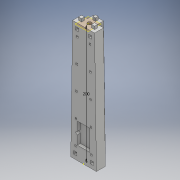
# Autodesk Inventor part: tb3_pt3
Saved by Autodesk Inventor 2017 (Build 210142000, 142)
## iProperties
Created: 2017-04-07
Part Number: tb3_pt3
Material: Generic
Document SubType Name: Modeling
Designer: PC
Density: 1 g/cm^3
Appearance: Default
Author: PC
Autodesk Inventor part; units mm, degrees
ref_plane "YZ Plane" through (0, 0, 0) normal (1, 0, 0) x (0, 1, 0)
ref_plane "XZ Plane" through (0, 0, 0) normal (0, 1, 0) x (-1, 0, 0)
ref_plane "XY Plane" through (0, 0, 0) normal (0, 0, 1) x (1, 0, 0)
sketch "Sketch1" plane through (0, 0, 0) normal (0, 0, 1) x (1, 0, 0)
  line L0 (21.5, -7.5) -> (-21.5, -7.5)
  line L1 (-21.5, -7.5) -> (-21.5, 7.5)
  line L2 (-21.5, 7.5) -> (21.5, 7.5)
  line L3 (21.5, 7.5) -> (21.5, -7.5)
  line L4 (21.5, -7.5) -> (-21.5, 7.5) construction
  line L5 (-21.5, -7.5) -> (21.5, 7.5) construction
  point P0 (0, 0)
  dimension "d0" = 43
  dimension "d1" = 15
  constraints: 12 end point, 2 midpoint, 2 parallel, 1 horizontal, 1 perpendicular
  measures "d0" distance of L1.end L2.end
  measures "d1" distance of L0.end L1.end
sketch "Sketch2" plane through (0, 0, 0) normal (0, 0, 1) x (1, 0, 0)
  line L0 (0, 0) -> (0, 12.5)
  line L1 (11.5, 17.5) -> (-11.5, 17.5)
  line L2 (-11.5, 17.5) -> (-11.5, 7.5)
  line L3 (-11.5, 7.5) -> (11.5, 7.5)
  line L4 (11.5, 7.5) -> (11.5, 17.5)
  line L5 (11.5, 17.5) -> (-11.5, 7.5) construction
  line L6 (-11.5, 17.5) -> (11.5, 7.5) construction
  dimension "d2" = 12.5
  dimension "d3" = 23
  dimension "d4" = 10
  constraints: 14 end point, 2 midpoint, 2 parallel, 1 horizontal, 1 perpendicular, 1 vertical
  measures "d2" distance of L0.start L0.end
  measures "d3" distance of L3.end L2.end
  measures "d4" distance of L2.end L1.end
sketch "Sketch3" plane through (0, 0, 0) normal (1, 0, 0) x (0, 1, 0)
  line L0 (0, 0) -> (0, 200)
  dimension "d5" = 200
  constraints: 2 end point, 1 vertical
  measures "d5" distance of L0.start L0.end
ref_plane "Work Plane1" through (0, 0, 200) normal (0, 0, 1) x (1, 0, 0)
sketch "Sketch4" plane through (0, 0, 200) normal (0, 0, 1) x (1, 0, 0)
  line L0 (18.5, -7.5) -> (-18.5, -7.5)
  line L1 (-18.5, -7.5) -> (-18.5, 7.5)
  line L2 (-18.5, 7.5) -> (18.5, 7.5)
  line L3 (18.5, 7.5) -> (18.5, -7.5)
  line L4 (18.5, -7.5) -> (-18.5, 7.5) construction
  line L5 (-18.5, -7.5) -> (18.5, 7.5) construction
  point P0 (0, 0)
  dimension "d6" = 37
  dimension "d7" = 15
  constraints: 12 end point, 2 midpoint, 2 parallel, 1 horizontal, 1 perpendicular
  measures "d6" distance of L1.end L2.end
  measures "d7" distance of L0.end L1.end
sketch "Sketch5" plane through (0, 0, 200) normal (0, 0, 1) x (1, 0, 0)
  line L0 (0, 0) -> (0, 12.5)
  line L1 (-8.5, 17.5) -> (8.5, 17.5)
  line L2 (8.5, 17.5) -> (8.5, 7.5)
  line L3 (8.5, 7.5) -> (-8.5, 7.5)
  line L4 (-8.5, 7.5) -> (-8.5, 17.5)
  line L5 (-8.5, 17.5) -> (8.5, 7.5) construction
  line L6 (8.5, 17.5) -> (-8.5, 7.5) construction
  dimension "d8" = 12.5
  dimension "d9" = 17
  dimension "d10" = 10
  constraints: 14 end point, 2 midpoint, 2 parallel, 1 horizontal, 1 perpendicular, 1 vertical
  measures "d8" distance of L0.start L0.end
  measures "d9" distance of L2.end L3.end
  measures "d10" distance of L1.end L2.end
loft "Loft1" add profiles "Sketch4", "Sketch1"
loft "Loft2" add profiles "Sketch5", "Sketch2"
sketch "Sketch7" plane through (21.5, -7.5, 0) normal (0, 0, -1) x (-1, 0, 0)
  line L0 (30, 25) -> (13, 25) projected
  line L1 (10, 15) -> (13, 15) projected
  line L2 (21.5, 25) -> (10, 25)
  line L3 (10, 25) -> (10, 15)
  line L4 (10, 15) -> (21.5, 15)
  line L5 (21.5, 15) -> (21.5, 25)
  line L6 (10, 25) -> (10, 15) projected
  line L7 (10, 25) -> (15.75, 25)
  line L8 (15.75, 25) -> (15.75, 15)
  line L9 (15.75, 15) -> (10, 15)
  line L10 (10, 15) -> (10, 25)
  line L11 (18.5, 17.25) -> (13, 17.25)
  line L12 (13, 17.25) -> (13, 22.75)
  line L13 (13, 22.75) -> (18.5, 22.75)
  line L14 (18.5, 22.75) -> (18.5, 17.25)
  line L15 (18.5, 17.25) -> (13, 22.75) construction
  line L16 (13, 17.25) -> (18.5, 22.75) construction
  point P0 (21.5, 7.5)
  point P1 (15.75, 20)
  dimension "d30" = 5.5
  dimension "d31" = 5.5
  constraints: 28 end point, 6 parallel, 5 midpoint, 3 horizontal, 3 perpendicular
  measures "d30" distance of L12.end L13.end
  measures "d31" distance of L11.end L12.end
sketch "Sketch8" plane through (21.5, -7.5, 0) normal (0, 0, -1) x (-1, 0, 0)
  line L0 (30, 25) -> (13, 25) projected
  line L1 (33, 15) -> (33, 25) projected
  line L2 (21.5, 25) -> (33, 25)
  line L3 (33, 25) -> (33, 15)
  line L4 (33, 15) -> (21.5, 15)
  line L5 (21.5, 15) -> (21.5, 25)
  line L6 (33, 25) -> (27.25, 25)
  line L7 (27.25, 25) -> (27.25, 15)
  line L8 (27.25, 15) -> (33, 15)
  line L9 (33, 15) -> (33, 25)
  line L10 (30, 17.25) -> (24.5, 17.25)
  line L11 (24.5, 17.25) -> (24.5, 22.75)
  line L12 (24.5, 22.75) -> (30, 22.75)
  line L13 (30, 22.75) -> (30, 17.25)
  line L14 (30, 17.25) -> (24.5, 22.75) construction
  line L15 (24.5, 17.25) -> (30, 22.75) construction
  point P0 (21.5, 7.5)
  point P1 (27.25, 20)
  dimension "d32" = 5.5
  dimension "d33" = 5.5
  constraints: 28 end point, 6 parallel, 5 midpoint, 3 horizontal, 3 perpendicular
  measures "d32" distance of L11.end L12.end
  measures "d33" distance of L10.end L11.end
extrude "Extrusion10" cut sketch "Sketch7" against normal blind 6 contours L13 L14 L11 L8 | L8 L11 L12 L13
extrude "Extrusion11" cut sketch "Sketch8" against normal blind 6 contours L12 L13 L10 L7 | L7 L10 L11 L12
sketch "Sketch15" plane through (8.5, 7.5, 200) normal (0, 1, 0) x (1, 0, 0)
  line L0 (0, 0) -> (3, 200) projected
  line L1 (2.6994, 179.9593) -> (4.6994, 179.9593)
  line L2 (2.6994, 179.9593) -> (4.6994, 179.9593) construction
  line L3 (4.0994, 180.5593) -> (5.2994, 180.5593)
  line L4 (5.2994, 180.5593) -> (5.2994, 179.3593)
  line L5 (5.2994, 179.3593) -> (4.0994, 179.3593)
  line L6 (4.0994, 179.3593) -> (4.0994, 180.5593)
  line L7 (4.0994, 180.5593) -> (5.2994, 179.3593) construction
  line L8 (5.2994, 180.5593) -> (4.0994, 179.3593) construction
  point P0 (-8.5, 200)
  dimension "d78" = 2
  dimension "d79" = 0
  dimension "d82" = 1.2
  dimension "d83" = 1.2
  constraints: 16 end point, 3 horizontal, 2 midpoint, 2 parallel, 1 collinear, 1 perpendicular, 1 point on line
  measures "d78" distance of L1.start L1.end
  measures "d79" distance between parallel lines of L1 L2
  measures "d82" distance of L4.end L5.end
  measures "d83" distance of L3.end L4.end
sketch "Sketch16" plane through (8.5, 7.5, 200) normal (0, 1, 0) x (1, 0, 0)
  line L0 (0, 0) -> (3, 200) projected
  line L1 (2.0995, 139.9683) -> (4.0995, 139.9683)
  line L2 (2.0995, 139.9683) -> (4.0995, 139.9683) construction
  line L3 (3.4995, 140.5683) -> (4.6995, 140.5683)
  line L4 (4.6995, 140.5683) -> (4.6995, 139.3683)
  line L5 (4.6995, 139.3683) -> (3.4995, 139.3683)
  line L6 (3.4995, 139.3683) -> (3.4995, 140.5683)
  line L7 (3.4995, 140.5683) -> (4.6995, 139.3683) construction
  line L8 (4.6995, 140.5683) -> (3.4995, 139.3683) construction
  point P0 (-8.5, 200)
  dimension "d80" = 2
  dimension "d81" = 0
  dimension "d95" = 1.2
  dimension "d96" = 1.2
  constraints: 16 end point, 3 horizontal, 2 midpoint, 2 parallel, 1 collinear, 1 perpendicular, 1 point on line
  measures "d80" distance of L1.start L1.end
  measures "d81" distance between parallel lines of L1 L2
  measures "d95" distance of L4.end L5.end
  measures "d96" distance of L3.end L4.end
sketch "Sketch18" plane through (8.5, 7.5, 200) normal (0, 1, 0) x (1, 0, 0)
  line L0 (3, 200) -> (0, 0) projected
  line L1 (1.5, 100) -> (3.5, 100)
  line L2 (2.9, 100.6) -> (4.1, 100.6)
  line L3 (4.1, 100.6) -> (4.1, 99.4)
  line L4 (4.1, 99.4) -> (2.9, 99.4)
  line L5 (2.9, 99.4) -> (2.9, 100.6)
  line L6 (2.9, 100.6) -> (4.1, 99.4) construction
  line L7 (4.1, 100.6) -> (2.9, 99.4) construction
  point P0 (-8.5, 200)
  dimension "d90" = 2
  dimension "d103" = 1.2
  dimension "d104" = 1.2
  constraints: 14 end point, 3 midpoint, 2 horizontal, 2 parallel, 1 perpendicular
  measures "d90" distance of L1.start L1.end
  measures "d103" distance of L3.end L4.end
  measures "d104" distance of L2.end L3.end
sketch "Sketch19" plane through (8.5, 7.5, 200) normal (0, 1, 0) x (1, 0, 0)
  line L0 (3, 200) -> (0, 0) projected
  line L1 (0.8998, 59.9862) -> (2.8998, 59.9862)
  line L2 (0.8998, 59.9862) -> (2.8998, 59.9862) construction
  line L3 (2.2998, 60.5862) -> (3.4998, 60.5862)
  line L4 (3.4998, 60.5862) -> (3.4998, 59.3862)
  line L5 (3.4998, 59.3862) -> (2.2998, 59.3862)
  line L6 (2.2998, 59.3862) -> (2.2998, 60.5862)
  line L7 (2.2998, 60.5862) -> (3.4998, 59.3862) construction
  line L8 (3.4998, 60.5862) -> (2.2998, 59.3862) construction
  point P0 (-8.5, 200)
  dimension "d91" = 2
  dimension "d92" = 0
  dimension "d111" = 1.2
  dimension "d112" = 1.2
  constraints: 16 end point, 3 horizontal, 2 midpoint, 2 parallel, 1 collinear, 1 perpendicular, 1 point on line
  measures "d91" distance of L1.start L1.end
  measures "d92" distance between parallel lines of L1 L2
  measures "d111" distance of L4.end L5.end
  measures "d112" distance of L3.end L4.end
sketch "Sketch20" plane through (8.5, 7.5, 200) normal (0, 1, 0) x (1, 0, 0)
  line L0 (3, 200) -> (0, 0) projected
  line L1 (0.2999, 19.9952) -> (2.2999, 19.9952)
  line L2 (0.2999, 19.9952) -> (2.2999, 19.9952) construction
  line L3 (1.6999, 20.5952) -> (2.8999, 20.5952)
  line L4 (2.8999, 20.5952) -> (2.8999, 19.3952)
  line L5 (2.8999, 19.3952) -> (1.6999, 19.3952)
  line L6 (1.6999, 19.3952) -> (1.6999, 20.5952)
  line L7 (1.6999, 20.5952) -> (2.8999, 19.3952) construction
  line L8 (2.8999, 20.5952) -> (1.6999, 19.3952) construction
  point P0 (-8.5, 200)
  dimension "d93" = 2
  dimension "d94" = 0
  dimension "d119" = 1.2
  dimension "d120" = 1.2
  constraints: 16 end point, 3 horizontal, 2 midpoint, 2 parallel, 1 collinear, 1 perpendicular, 1 point on line
  measures "d93" distance of L1.start L1.end
  measures "d94" distance between parallel lines of L1 L2
  measures "d119" distance of L4.end L5.end
  measures "d120" distance of L3.end L4.end
extrude "Extrusion17" cut sketch "Sketch15" against normal blind 6.6
sketch "Sketch17" plane through (8.5, 0.9, 200) normal (0, 1, 0) x (1, 0, 0)
  line L0 (3.3, 181.4) -> (6.1, 181.4)
  line L1 (6.1, 181.4) -> (6.1, 178.6)
  line L2 (6.1, 178.6) -> (3.3, 178.6)
  line L3 (3.3, 178.6) -> (3.3, 181.4)
  line L4 (3.3, 181.4) -> (6.1, 178.6) construction
  line L5 (6.1, 181.4) -> (3.3, 178.6) construction
  point P0 (-8.5, 200)
  point P1 (4.7, 180)
  dimension "d86" = 2.8
  dimension "d87" = 2.8
  constraints: 12 end point, 2 midpoint, 2 parallel, 1 horizontal, 1 perpendicular
  measures "d86" distance of L1.end L2.end
  measures "d87" distance of L0.end L1.end
extrude "Extrusion18" cut sketch "Sketch17" against normal through all
extrude "Extrusion19" cut sketch "Sketch16" against normal blind 6.6
sketch "Sketch21" plane through (8.5, 0.9, 200) normal (0, 1, 0) x (1, 0, 0)
  line L0 (2.7, 141.4) -> (5.5, 141.4)
  line L1 (5.5, 141.4) -> (5.5, 138.6)
  line L2 (5.5, 138.6) -> (2.7, 138.6)
  line L3 (2.7, 138.6) -> (2.7, 141.4)
  line L4 (2.7, 141.4) -> (5.5, 138.6) construction
  line L5 (5.5, 141.4) -> (2.7, 138.6) construction
  point P0 (-8.5, 200)
  point P1 (4.1, 140)
  dimension "d99" = 2.8
  dimension "d100" = 2.8
  constraints: 12 end point, 2 midpoint, 2 parallel, 1 horizontal, 1 perpendicular
  measures "d99" distance of L1.end L2.end
  measures "d100" distance of L0.end L1.end
extrude "Extrusion20" cut sketch "Sketch21" against normal through all
extrude "Extrusion21" cut sketch "Sketch18" against normal blind 6.6
sketch "Sketch22" plane through (8.5, 0.9, 200) normal (0, 1, 0) x (1, 0, 0)
  line L0 (2.1, 101.4) -> (4.9, 101.4)
  line L1 (4.9, 101.4) -> (4.9, 98.6)
  line L2 (4.9, 98.6) -> (2.1, 98.6)
  line L3 (2.1, 98.6) -> (2.1, 101.4)
  line L4 (2.1, 101.4) -> (4.9, 98.6) construction
  line L5 (4.9, 101.4) -> (2.1, 98.6) construction
  point P0 (-8.5, 200)
  point P1 (3.5, 100)
  dimension "d107" = 2.8
  dimension "d108" = 2.8
  constraints: 12 end point, 2 midpoint, 2 parallel, 1 horizontal, 1 perpendicular
  measures "d107" distance of L1.end L2.end
  measures "d108" distance of L0.end L1.end
extrude "Extrusion22" cut sketch "Sketch22" against normal through all
extrude "Extrusion23" cut sketch "Sketch19" against normal blind 6.6
sketch "Sketch23" plane through (8.5, 0.9, 200) normal (0, 1, 0) x (1, 0, 0)
  line L0 (1.5, 61.4) -> (4.3, 61.4)
  line L1 (4.3, 61.4) -> (4.3, 58.6)
  line L2 (4.3, 58.6) -> (1.5, 58.6)
  line L3 (1.5, 58.6) -> (1.5, 61.4)
  line L4 (1.5, 61.4) -> (4.3, 58.6) construction
  line L5 (4.3, 61.4) -> (1.5, 58.6) construction
  point P0 (-8.5, 200)
  point P1 (2.9, 60)
  dimension "d115" = 2.8
  dimension "d116" = 2.8
  constraints: 12 end point, 2 midpoint, 2 parallel, 1 horizontal, 1 perpendicular
  measures "d115" distance of L1.end L2.end
  measures "d116" distance of L0.end L1.end
extrude "Extrusion24" cut sketch "Sketch23" against normal through all
extrude "Extrusion25" cut sketch "Sketch20" against normal blind 6.6
sketch "Sketch24" plane through (8.5, 0.9, 200) normal (0, 1, 0) x (1, 0, 0)
  line L0 (0.9, 21.4) -> (3.7, 21.4)
  line L1 (3.7, 21.4) -> (3.7, 18.6)
  line L2 (3.7, 18.6) -> (0.9, 18.6)
  line L3 (0.9, 18.6) -> (0.9, 21.4)
  line L4 (0.9, 21.4) -> (3.7, 18.6) construction
  line L5 (3.7, 21.4) -> (0.9, 18.6) construction
  point P0 (-8.5, 200)
  point P1 (2.3, 20)
  dimension "d123" = 2.8
  dimension "d124" = 2.8
  constraints: 12 end point, 2 midpoint, 2 parallel, 1 horizontal, 1 perpendicular
  measures "d123" distance of L1.end L2.end
  measures "d124" distance of L0.end L1.end
extrude "Extrusion26" cut sketch "Sketch24" against normal through all
sketch "Sketch26" plane through (-21.5, 7.5, 0) normal (0, 1, 0) x (1, 0, 0)
  line L0 (13, -200) -> (10, 0) projected
  line L1 (10.3, -20) -> (8.3, -20)
  line L2 (10.3, -20) -> (12.3, -20) construction
  line L3 (7.7, -19.4) -> (8.9, -19.4)
  line L4 (8.9, -19.4) -> (8.9, -20.6)
  line L5 (8.9, -20.6) -> (7.7, -20.6)
  line L6 (7.7, -20.6) -> (7.7, -19.4)
  line L7 (7.7, -19.4) -> (8.9, -20.6) construction
  line L8 (8.9, -19.4) -> (7.7, -20.6) construction
  point P0 (21.5, 0)
  dimension "d127" = 2
  dimension "d128" = 180
  dimension "d129" = 1.2
  dimension "d130" = 1.2
  constraints: 16 end point, 3 horizontal, 2 midpoint, 2 parallel, 1 collinear, 1 perpendicular, 1 point on line
  measures "d127" distance of L1.start L1.end
  measures "d128" angle of L1 L2
  measures "d129" distance of L4.end L5.end
  measures "d130" distance of L3.end L4.end
extrude "Extrusion27" cut sketch "Sketch26" against normal blind 6.6
sketch "Sketch27" plane through (-21.5, 0.9, 0) normal (0, 1, 0) x (1, 0, 0)
  line L0 (6.9, -18.6) -> (9.7, -18.6)
  line L1 (9.7, -18.6) -> (9.7, -21.4)
  line L2 (9.7, -21.4) -> (6.9, -21.4)
  line L3 (6.9, -21.4) -> (6.9, -18.6)
  line L4 (6.9, -18.6) -> (9.7, -21.4) construction
  line L5 (9.7, -18.6) -> (6.9, -21.4) construction
  point P0 (21.5, 0)
  point P1 (8.3, -20)
  dimension "d133" = 2.8
  dimension "d134" = 2.8
  constraints: 12 end point, 2 midpoint, 2 parallel, 1 horizontal, 1 perpendicular
  measures "d133" distance of L1.end L2.end
  measures "d134" distance of L0.end L1.end
extrude "Extrusion28" cut sketch "Sketch27" against normal through all
sketch "Sketch28" plane through (-21.5, 7.5, 0) normal (0, 1, 0) x (1, 0, 0)
  line L0 (13, -200) -> (10, 0) projected
  line L1 (10.9, -60) -> (8.9, -60)
  line L2 (10.9, -60) -> (12.9, -60) construction
  line L3 (8.3, -59.4) -> (9.5, -59.4)
  line L4 (9.5, -59.4) -> (9.5, -60.6)
  line L5 (9.5, -60.6) -> (8.3, -60.6)
  line L6 (8.3, -60.6) -> (8.3, -59.4)
  line L7 (8.3, -59.4) -> (9.5, -60.6) construction
  line L8 (9.5, -59.4) -> (8.3, -60.6) construction
  point P0 (21.5, 0)
  dimension "d137" = 2
  dimension "d138" = 180
  dimension "d139" = 1.2
  dimension "d140" = 1.2
  constraints: 16 end point, 3 horizontal, 2 midpoint, 2 parallel, 1 collinear, 1 perpendicular, 1 point on line
  measures "d137" distance of L1.start L1.end
  measures "d138" angle of L1 L2
  measures "d139" distance of L4.end L5.end
  measures "d140" distance of L3.end L4.end
extrude "Extrusion29" cut sketch "Sketch28" against normal blind 6.6
sketch "Sketch29" plane through (-21.5, 0.9, 0) normal (0, 1, 0) x (1, 0, 0)
  line L0 (7.5, -58.6) -> (10.3, -58.6)
  line L1 (10.3, -58.6) -> (10.3, -61.4)
  line L2 (10.3, -61.4) -> (7.5, -61.4)
  line L3 (7.5, -61.4) -> (7.5, -58.6)
  line L4 (7.5, -58.6) -> (10.3, -61.4) construction
  line L5 (10.3, -58.6) -> (7.5, -61.4) construction
  point P0 (21.5, 0)
  point P1 (8.9, -60)
  dimension "d143" = 2.8
  dimension "d144" = 2.8
  constraints: 12 end point, 2 midpoint, 2 parallel, 1 horizontal, 1 perpendicular
  measures "d143" distance of L1.end L2.end
  measures "d144" distance of L0.end L1.end
extrude "Extrusion30" cut sketch "Sketch29" against normal through all
sketch "Sketch30" plane through (-21.5, 7.5, 0) normal (0, 1, 0) x (1, 0, 0)
  line L0 (13, -200) -> (10, 0) projected
  line L1 (11.5, -100) -> (9.5, -100)
  line L2 (10.1, -99.4) -> (8.9, -99.4)
  line L3 (8.9, -99.4) -> (8.9, -100.6)
  line L4 (8.9, -100.6) -> (10.1, -100.6)
  line L5 (10.1, -100.6) -> (10.1, -99.4)
  line L6 (10.1, -99.4) -> (8.9, -100.6) construction
  line L7 (8.9, -99.4) -> (10.1, -100.6) construction
  point P0 (21.5, 0)
  dimension "d147" = 2
  dimension "d148" = 1.2
  dimension "d149" = 1.2
  constraints: 14 end point, 3 midpoint, 2 horizontal, 2 parallel, 1 perpendicular
  measures "d147" distance of L1.start L1.end
  measures "d148" distance of L4.end L3.end
  measures "d149" distance of L3.end L2.end
extrude "Extrusion31" cut sketch "Sketch30" against normal blind 6.6
sketch "Sketch31" plane through (-21.5, 0.9, 0) normal (0, 1, 0) x (1, 0, 0)
  line L0 (8.1, -98.6) -> (10.9, -98.6)
  line L1 (10.9, -98.6) -> (10.9, -101.4)
  line L2 (10.9, -101.4) -> (8.1, -101.4)
  line L3 (8.1, -101.4) -> (8.1, -98.6)
  line L4 (8.1, -98.6) -> (10.9, -101.4) construction
  line L5 (10.9, -98.6) -> (8.1, -101.4) construction
  point P0 (21.5, 0)
  point P1 (9.5, -100)
  dimension "d152" = 2.8
  dimension "d153" = 2.8
  constraints: 12 end point, 2 midpoint, 2 parallel, 1 horizontal, 1 perpendicular
  measures "d152" distance of L1.end L2.end
  measures "d153" distance of L0.end L1.end
extrude "Extrusion32" cut sketch "Sketch31" against normal through all
sketch "Sketch32" plane through (-21.5, 7.5, 0) normal (0, 1, 0) x (1, 0, 0)
  line L0 (13, -200) -> (10, 0) projected
  line L1 (12.1, -140) -> (10.1, -140)
  line L2 (12.1, -140) -> (14.1, -140) construction
  line L3 (10.7, -139.4) -> (9.5, -139.4)
  line L4 (9.5, -139.4) -> (9.5, -140.6)
  line L5 (9.5, -140.6) -> (10.7, -140.6)
  line L6 (10.7, -140.6) -> (10.7, -139.4)
  line L7 (10.7, -139.4) -> (9.5, -140.6) construction
  line L8 (9.5, -139.4) -> (10.7, -140.6) construction
  point P0 (21.5, 0)
  dimension "d156" = 2
  dimension "d157" = 180
  dimension "d158" = 1.2
  dimension "d159" = 1.2
  constraints: 16 end point, 3 horizontal, 2 midpoint, 2 parallel, 1 collinear, 1 perpendicular, 1 point on line
  measures "d156" distance of L1.start L1.end
  measures "d157" angle of L1 L2
  measures "d158" distance of L5.end L4.end
  measures "d159" distance of L4.end L3.end
extrude "Extrusion33" cut sketch "Sketch32" against normal blind 6.6
sketch "Sketch33" plane through (-21.5, 0.9, 0) normal (0, 1, 0) x (1, 0, 0)
  line L0 (8.7, -138.6) -> (11.5, -138.6)
  line L1 (11.5, -138.6) -> (11.5, -141.4)
  line L2 (11.5, -141.4) -> (8.7, -141.4)
  line L3 (8.7, -141.4) -> (8.7, -138.6)
  line L4 (8.7, -138.6) -> (11.5, -141.4) construction
  line L5 (11.5, -138.6) -> (8.7, -141.4) construction
  point P0 (21.5, 0)
  point P1 (10.1, -140)
  dimension "d162" = 2.8
  dimension "d163" = 2.8
  constraints: 12 end point, 2 midpoint, 2 parallel, 1 horizontal, 1 perpendicular
  measures "d162" distance of L1.end L2.end
  measures "d163" distance of L0.end L1.end
extrude "Extrusion34" cut sketch "Sketch33" against normal through all
sketch "Sketch34" plane through (-21.5, 7.5, 0) normal (0, 1, 0) x (1, 0, 0)
  line L0 (13, -200) -> (10, 0) projected
  line L1 (12.7, -180) -> (10.7, -180)
  line L2 (12.7, -180) -> (14.7, -180) construction
  line L3 (10.1, -179.4) -> (11.3, -179.4)
  line L4 (11.3, -179.4) -> (11.3, -180.6)
  line L5 (11.3, -180.6) -> (10.1, -180.6)
  line L6 (10.1, -180.6) -> (10.1, -179.4)
  line L7 (10.1, -179.4) -> (11.3, -180.6) construction
  line L8 (11.3, -179.4) -> (10.1, -180.6) construction
  point P0 (21.5, 0)
  dimension "d166" = 2
  dimension "d167" = 180
  dimension "d168" = 1.2
  dimension "d169" = 1.2
  constraints: 16 end point, 3 horizontal, 2 midpoint, 2 parallel, 1 collinear, 1 perpendicular, 1 point on line
  measures "d166" distance of L1.start L1.end
  measures "d167" angle of L1 L2
  measures "d168" distance of L4.end L5.end
  measures "d169" distance of L3.end L4.end
extrude "Extrusion35" cut sketch "Sketch34" against normal blind 6.6
sketch "Sketch35" plane through (-21.5, 0.9, 0) normal (0, 1, 0) x (1, 0, 0)
  line L0 (9.3, -178.6) -> (12.1, -178.6)
  line L1 (12.1, -178.6) -> (12.1, -181.4)
  line L2 (12.1, -181.4) -> (9.3, -181.4)
  line L3 (9.3, -181.4) -> (9.3, -178.6)
  line L4 (9.3, -178.6) -> (12.1, -181.4) construction
  line L5 (12.1, -178.6) -> (9.3, -181.4) construction
  point P0 (21.5, 0)
  point P1 (10.7, -180)
  dimension "d172" = 2.8
  dimension "d173" = 2.8
  constraints: 12 end point, 2 midpoint, 2 parallel, 1 horizontal, 1 perpendicular
  measures "d172" distance of L1.end L2.end
  measures "d173" distance of L0.end L1.end
extrude "Extrusion36" cut sketch "Sketch35" against normal through all
chamfer "Chamfer1" distance 0.8 angle 45 4 edges at (-13.8, 0.9, 20) (-13.2, 0.9, 20.6) (-12.6, 0.9, 20) (-13.2, 0.9, 19.4)
chamfer "Chamfer2" distance 0.8 angle 45 4 edges at (-13.2, 0.9, 60) (-12.6, 0.9, 60.6) (-12, 0.9, 60) (-12.6, 0.9, 59.4)
chamfer "Chamfer3" distance 0.8 angle 45 4 edges at (-12, 0.9, 100.6) (-12.6, 0.9, 100) (-12, 0.9, 99.4) (-11.4, 0.9, 100)
chamfer "Chamfer4" distance 0.8 angle 45 4 edges at (-12, 0.9, 140) (-11.4, 0.9, 140.6) (-10.8, 0.9, 140) (-11.4, 0.9, 139.4)
chamfer "Chamfer5" distance 0.8 angle 45 4 edges at (-10.8, 0.9, 180.6) (-11.4, 0.9, 180) (-10.8, 0.9, 179.4) (-10.2, 0.9, 180)
chamfer "Chamfer6" distance 0.73 angle 45 4 edges at (13.1994, 0.9, 19.4407) (12.5994, 0.9, 20.0407) (13.1994, 0.9, 20.6407) (13.7994, 0.9, 20.0407)
chamfer "Chamfer7" distance 0.7 angle 45 4 edges at (11.9995, 0.9, 60.0317) (12.5995, 0.9, 60.6317) (13.1995, 0.9, 60.0317) (12.5995, 0.9, 59.4317)
chamfer "Chamfer8" distance 0.8 angle 45 4 edges at (11.4, 0.9, 100) (12, 0.9, 100.6) (12.6, 0.9, 100) (12, 0.9, 99.4)
chamfer "Chamfer9" distance 0.7 angle 45 4 edges at (10.7998, 0.9, 140.0138) (11.3998, 0.9, 140.6138) (11.9998, 0.9, 140.0138) (11.3998, 0.9, 139.4138)
chamfer "Chamfer10" distance 0.7 angle 45 4 edges at (10.1999, 0.9, 180.0048) (10.7999, 0.9, 180.6048) (11.3999, 0.9, 180.0048) (10.7999, 0.9, 179.4048)
sketch "Sketch36" plane through (-18.5, -7.5, 200) normal (0, 0, 1) x (1, 0, 0)
  line L0 (7, 25) -> (30, 25) projected
  line L1 (18.5, 25) -> (18.5, 10)
  point P0 (18.5, 7.5)
  dimension "d206" = 15
  constraints: 2 end point, 1 midpoint, 1 vertical
  measures "d206" distance of L1.start L1.end
hole "Hole2" at (0, 2.5, 200) direction (0, 0, -1) diameter 6.4 end through all
sketch "Sketch37" plane through (-21.5, -7.5, 0) normal (0, -1, 0) x (1, 0, 0)
  point P0 (21.5, 0)
sketch "Sketch38" plane through (-21.5, -7.5, 0) normal (0, -1, 0) x (1, 0, 0)
  line L0 (0, 0) -> (7.5, 0)
  line L1 (7.5, 0) -> (7.5, 9)
  line L2 (7.5, 9) -> (0, 9)
  line L3 (0, 9) -> (0, 0)
  line L4 (10, 6.5) -> (5, 6.5)
  line L5 (5, 6.5) -> (5, 11.5)
  line L6 (5, 11.5) -> (10, 11.5)
  line L7 (10, 11.5) -> (10, 6.5)
  line L8 (10, 6.5) -> (5, 11.5) construction
  line L9 (5, 6.5) -> (10, 11.5) construction
  point P0 (21.5, 0)
  dimension "d214" = 7.5
  dimension "d215" = 9
  dimension "d216" = 5
  dimension "d217" = 5
  constraints: 20 end point, 4 parallel, 2 horizontal, 2 midpoint, 2 perpendicular
  measures "d214" distance of L2.end L1.end
  measures "d215" distance of L1.end L0.end
  measures "d216" distance of L5.end L6.end
  measures "d217" distance of L4.end L5.end
sketch "Sketch39" plane through (-21.5, -7.5, 0) normal (0, -1, 0) x (1, 0, 0)
  line L0 (43, 0) -> (35.5, 0)
  line L1 (35.5, 0) -> (35.5, 9)
  line L2 (35.5, 9) -> (43, 9)
  line L3 (43, 9) -> (43, 0)
  line L4 (33, 11.5) -> (38, 11.5)
  line L5 (38, 11.5) -> (38, 6.5)
  line L6 (38, 6.5) -> (33, 6.5)
  line L7 (33, 6.5) -> (33, 11.5)
  line L8 (33, 11.5) -> (38, 6.5) construction
  line L9 (38, 11.5) -> (33, 6.5) construction
  point P0 (21.5, 0)
  dimension "d218" = 7.5
  dimension "d219" = 9
  dimension "d220" = 5
  dimension "d221" = 5
  constraints: 20 end point, 4 parallel, 2 horizontal, 2 midpoint, 2 perpendicular
  measures "d218" distance of L1.end L2.end
  measures "d219" distance of L0.end L1.end
  measures "d220" distance of L5.end L6.end
  measures "d221" distance of L4.end L5.end
sketch "Sketch40" plane through (-21.5, -7.5, 0) normal (0, -1, 0) x (1, 0, 0)
  line L0 (3, 200) -> (13, 200) projected
  line L1 (3, 200) -> (10.5, 200)
  line L2 (10.5, 200) -> (10.5, 191)
  line L3 (10.5, 191) -> (3, 191)
  line L4 (3, 191) -> (3, 200)
  line L5 (13, 188.5) -> (8, 188.5)
  line L6 (8, 188.5) -> (8, 193.5)
  line L7 (8, 193.5) -> (13, 193.5)
  line L8 (13, 193.5) -> (13, 188.5)
  line L9 (13, 188.5) -> (8, 193.5) construction
  line L10 (8, 188.5) -> (13, 193.5) construction
  point P0 (21.5, 0)
  dimension "d222" = 7.5
  dimension "d223" = 9
  dimension "d224" = 5
  dimension "d225" = 5
  constraints: 20 end point, 4 parallel, 2 horizontal, 2 midpoint, 2 perpendicular
  measures "d222" distance of L2.end L3.end
  measures "d223" distance of L1.end L2.end
  measures "d224" distance of L6.end L7.end
  measures "d225" distance of L5.end L6.end
sketch "Sketch41" plane through (-21.5, -7.5, 0) normal (0, -1, 0) x (1, 0, 0)
  line L0 (40, 200) -> (43, 0) projected
  line L1 (40, 200) -> (32.5, 200)
  line L2 (32.5, 200) -> (32.5, 191)
  line L3 (32.5, 191) -> (40, 191)
  line L4 (40, 191) -> (40, 200)
  line L5 (30, 188.5) -> (35, 188.5)
  line L6 (35, 188.5) -> (35, 193.5)
  line L7 (35, 193.5) -> (30, 193.5)
  line L8 (30, 193.5) -> (30, 188.5)
  line L9 (30, 188.5) -> (35, 193.5) construction
  line L10 (35, 188.5) -> (30, 193.5) construction
  point P0 (21.5, 0)
  dimension "d226" = 7.5
  dimension "d227" = 9
  dimension "d228" = 5
  dimension "d229" = 5
  constraints: 20 end point, 4 parallel, 2 horizontal, 2 midpoint, 2 perpendicular
  measures "d226" distance of L3.end L2.end
  measures "d227" distance of L2.end L1.end
  measures "d228" distance of L7.end L6.end
  measures "d229" distance of L6.end L5.end
extrude "Extrusion37" cut sketch "Sketch38" against normal blind 6 contours L4 L5 L2 L1 | L1 L2 L5 L6 L7 L4
extrude "Extrusion38" cut sketch "Sketch39" against normal blind 6 contours L6 L7 L4 L5 L2 L1 | L1 L2 L5 L6
extrude "Extrusion39" cut sketch "Sketch40" against normal blind 6 contours L7 L8 L5 L6 L3 L2 | L2 L3 L6 L7
extrude "Extrusion40" cut sketch "Sketch41" against normal blind 6 contours L7 L6 L3 L2 | L2 L3 L6 L5 L8 L7
sketch "Sketch42" plane through (-18.5, -7.5, 200) normal (0, 0, 1) x (1, 0, 0)
  line L0 (27, 25) -> (27, 15) projected
  line L1 (10, 15) -> (10, 25) projected
  line L2 (27, 15) -> (10, 15)
  line L3 (10, 15) -> (10, 25)
  line L4 (10, 25) -> (27, 25)
  line L5 (27, 25) -> (27, 15)
  line L6 (10, 25) -> (27, 25)
  line L7 (27, 25) -> (27, 20)
  line L8 (27, 20) -> (10, 20)
  line L9 (10, 20) -> (10, 25)
  line L10 (16.25, 22.25) -> (20.75, 22.25)
  line L11 (20.75, 22.25) -> (20.75, 17.75)
  line L12 (20.75, 17.75) -> (16.25, 17.75)
  line L13 (16.25, 17.75) -> (16.25, 22.25)
  line L14 (16.25, 22.25) -> (20.75, 17.75) construction
  line L15 (20.75, 22.25) -> (16.25, 17.75) construction
  point P0 (18.5, 7.5)
  point P1 (18.5, 20)
  dimension "d238" = 4.5
  dimension "d239" = 4.5
  constraints: 28 end point, 6 parallel, 4 midpoint, 3 horizontal, 3 perpendicular
  measures "d238" distance of L11.end L12.end
  measures "d239" distance of L10.end L11.end
extrude "Extrusion41" add sketch "Sketch42" along normal blind 5 contours L11 L12 L13 L8 | L8 L13 L10 L11
sketch "Sketch43" plane through (-21.5, -7.5, 0) normal (0, -1, 0) x (1, 0, 0)
  line L0 (32, 57.5) -> (11, 57.5)
  line L1 (11, 57.5) -> (11, 22.5)
  line L2 (11, 22.5) -> (32, 22.5)
  line L3 (32, 22.5) -> (32, 57.5)
  line L4 (32, 57.5) -> (11, 22.5) construction
  line L5 (11, 57.5) -> (32, 22.5) construction
  point P0 (21.5, 0)
  point P1 (21.5, 40)
  dimension "d242" = 21
  dimension "d243" = 35
  constraints: 12 end point, 2 midpoint, 2 parallel, 1 horizontal, 1 perpendicular
  measures "d242" distance of L2.end L1.end
  measures "d243" distance of L1.end L0.end
extrude "Extrusion42" cut sketch "Sketch43" against normal blind 5
sketch "Sketch44" plane through (-21.5, -7.5, 0) normal (0, -1, 0) x (1, 0, 0)
  line L0 (11, 22.5) -> (11, 57.5) projected
  circle A0 centre (11, 40) radius 2.5
  point P0 (21.5, 0)
  dimension "d246" = 5
  constraints: 1 centre point, 1 midpoint
  measures "d246" diameter of A0
extrude "Extrusion43" cut sketch "Sketch44" against normal blind 5
sketch "Sketch45" plane through (-18.5, -7.5, 200) normal (0, 0, 1) x (1, 0, 0)
  line L0 (0, 0) -> (0, 15) projected
  line L1 (0, 0) -> (5, 0)
  line L2 (5, 0) -> (5, 5)
  line L3 (5, 5) -> (0, 5)
  line L4 (0, 5) -> (0, 0)
  line L5 (5, 5) -> (10, 5)
  line L6 (10, 5) -> (10, 10)
  line L7 (10, 10) -> (5, 10)
  line L8 (5, 10) -> (5, 5)
  point P0 (18.5, 7.5)
  dimension "d249" = 5
  dimension "d250" = 5
  dimension "d251" = 5
  dimension "d252" = 5
  constraints: 16 end point, 4 parallel, 2 horizontal, 2 perpendicular
  measures "d249" distance of L3.end L2.end
  measures "d250" distance of L2.end L1.end
  measures "d251" distance of L7.end L6.end
  measures "d252" distance of L6.end L5.end
sketch "Sketch47" plane through (-18.5, -7.5, 200) normal (0, 0, 1) x (1, 0, 0)
  point P0 (18.5, 7.5)
extrude "Extrusion44" add sketch "Sketch45" along normal blind 5 contours L8 L7 L6 L5
sketch "Sketch48" plane through (-18.5, -7.5, 200) normal (0, 0, 1) x (1, 0, 0)
  line L0 (37, 15) -> (37, 0) projected
  line L1 (37, 0) -> (32, 0)
  line L2 (32, 0) -> (32, 5)
  line L3 (32, 5) -> (37, 5)
  line L4 (37, 5) -> (37, 0)
  line L5 (32, 5) -> (27, 5)
  line L6 (27, 5) -> (27, 10)
  line L7 (27, 10) -> (32, 10)
  line L8 (32, 10) -> (32, 5)
  point P0 (18.5, 7.5)
  dimension "d255" = 5
  dimension "d256" = 5
  dimension "d257" = 5
  dimension "d258" = 5
  constraints: 16 end point, 4 parallel, 2 horizontal, 2 perpendicular
  measures "d255" distance of L2.end L3.end
  measures "d256" distance of L1.end L2.end
  measures "d257" distance of L6.end L7.end
  measures "d258" distance of L5.end L6.end
extrude "Extrusion45" add sketch "Sketch48" along normal blind 5 contours L5 L6 L7 L8
sketch "Sketch49" plane through (21.5, -7.5, 0) normal (0, 0, -1) x (-1, 0, 0)
  line L0 (0, 15) -> (0, 0) projected
  line L1 (0, 0) -> (4.75, 0)
  line L2 (4.75, 0) -> (4.75, 4.75)
  line L3 (4.75, 4.75) -> (0, 4.75)
  line L4 (0, 4.75) -> (0, 0)
  line L5 (4.75, 4.75) -> (10.25, 4.75)
  line L6 (10.25, 4.75) -> (10.25, 10.25)
  line L7 (10.25, 10.25) -> (4.75, 10.25)
  line L8 (4.75, 10.25) -> (4.75, 4.75)
  point P0 (21.5, 7.5)
  dimension "d261" = 4.75
  dimension "d262" = 4.75
  dimension "d263" = 5.5
  dimension "d264" = 5.5
  constraints: 16 end point, 4 parallel, 2 horizontal, 2 perpendicular
  measures "d261" distance of L3.end L2.end
  measures "d262" distance of L2.end L1.end
  measures "d263" distance of L7.end L6.end
  measures "d264" distance of L6.end L5.end
extrude "Extrusion46" cut sketch "Sketch49" against normal blind 6 contours L8 L7 L6 L5
sketch "Sketch50" plane through (21.5, -7.5, 0) normal (0, 0, -1) x (-1, 0, 0)
  line L0 (40, 0) -> (43, 0) projected
  line L1 (43, 0) -> (38.25, 0)
  line L2 (38.25, 0) -> (38.25, 4.75)
  line L3 (38.25, 4.75) -> (43, 4.75)
  line L4 (43, 4.75) -> (43, 0)
  line L5 (38.25, 4.75) -> (32.75, 4.75)
  line L6 (32.75, 4.75) -> (32.75, 10.25)
  line L7 (32.75, 10.25) -> (38.25, 10.25)
  line L8 (38.25, 10.25) -> (38.25, 4.75)
  point P0 (21.5, 7.5)
  dimension "d267" = 4.75
  dimension "d268" = 4.75
  dimension "d269" = 5.5
  dimension "d270" = 5.5
  constraints: 16 end point, 4 parallel, 2 horizontal, 2 perpendicular
  measures "d267" distance of L2.end L3.end
  measures "d268" distance of L1.end L2.end
  measures "d269" distance of L6.end L7.end
  measures "d270" distance of L5.end L6.end
extrude "Extrusion47" cut sketch "Sketch50" against normal blind 6 contours L5 L6 L7 L8
body "Solid1"
